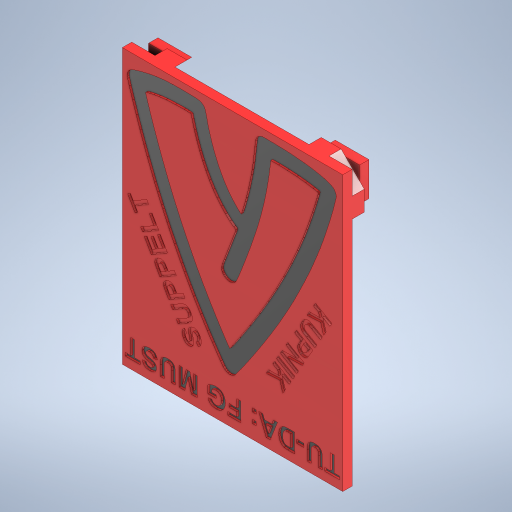
# Autodesk Inventor part: Battery_Cover
Saved by Autodesk Inventor 2023.3 (Build 273359000, 359)
## iProperties
Created: 2024-05-31
Part Number: Battery_Cover
Material: Generic
Document SubType Name: Modeling
Designer: Sven
Density: 1 g/cm^3
Appearance: Light Red
Author: Sven
Autodesk Inventor part; units mm, degrees
ref_plane "YZ Plane" through (0, 0, 0) normal (1, 0, 0) x (0, 1, 0)
ref_plane "XZ Plane" through (0, 0, 0) normal (0, 1, 0) x (-1, 0, 0)
ref_plane "XY Plane" through (0, 0, 0) normal (0, 0, 1) x (1, 0, 0)
sketch "Sketch1" plane through (0, 0, 0) normal (0, 0, 1) x (1, 0, 0)
  line L0 (1.45, 1.25) -> (1.45, -57.25) projected
  arc A0 (1.25, -57.45) -> (1.45, -57.25) centre (1.25, -57.25) ccw projected
  line L1 (1.25, -57.45) -> (-45.75, -57.45) projected
  arc A1 (-45.95, -57.25) -> (-45.75, -57.45) centre (-45.75, -57.25) ccw projected
  line L2 (-45.95, -57.25) -> (-45.95, 1.25) projected
  arc A2 (-45.75, 1.45) -> (-45.95, 1.25) centre (-45.75, 1.25) ccw projected
  line L3 (-45.75, 1.45) -> (1.25, 1.45) projected
  arc A3 (1.45, 1.25) -> (1.25, 1.45) centre (1.25, 1.25) ccw projected
  arc A4 (-45.75, 3.25) -> (-47.75, 1.25) centre (-45.75, 1.25) ccw projected
  line L4 (-47.75, -57.25) -> (-47.75, 1.25) projected
  arc A5 (-47.75, -57.25) -> (-45.75, -59.25) centre (-45.75, -57.25) ccw projected
  line L5 (1.25, -59.25) -> (-45.75, -59.25) projected
  arc A6 (1.25, -59.25) -> (3.25, -57.25) centre (1.25, -57.25) ccw projected
  line L6 (3.25, 1.25) -> (3.25, -57.25) projected
  arc A7 (3.25, 1.25) -> (1.25, 3.25) centre (1.25, 1.25) ccw projected
  line L7 (-45.75, 3.25) -> (1.25, 3.25) projected
  line L8 (1.25, 1.25) -> (-45.75, 1.25)
  line L9 (-45.75, 1.25) -> (-45.75, -57.25)
  line L10 (-45.75, -57.25) -> (1.25, -57.25)
  line L11 (1.25, -57.25) -> (1.25, 1.25)
  point P0 (0, 0)
  dimension "d0" = 0.2
  constraints: 8 end point, 23 other
  measures "d0" radius of A3
extrude "Extrusion1" add sketch "Sketch1" along normal blind 2 contours L11 L10 L9 L8
sketch "Sketch2" plane through (0, 0, 0) normal (0, 0, -1) x (-1, 0, 0)
  line L0 (-1.45, -3.05) -> (3.05, 1.45) projected
  line L1 (41.45, 1.45) -> (45.95, -3.05) projected
  line L2 (-1.45, 1.25) -> (-1.45, -57.25) projected
  arc A0 (-1.45, -57.25) -> (-1.25, -57.45) centre (-1.25, -57.25) ccw projected
  line L3 (-1.25, -57.45) -> (45.75, -57.45) projected
  arc A1 (45.75, -57.45) -> (45.95, -57.25) centre (45.75, -57.25) ccw projected
  line L4 (45.95, -57.25) -> (45.95, 1.25) projected
  arc A2 (45.95, 1.25) -> (45.75, 1.45) centre (45.75, 1.25) ccw projected
  line L5 (45.75, 1.45) -> (-1.25, 1.45) projected
  arc A3 (-1.25, 1.45) -> (-1.45, 1.25) centre (-1.25, 1.25) ccw projected
  arc A4 (47.75, 1.25) -> (45.75, 3.25) centre (45.75, 1.25) ccw projected
  line L6 (47.75, -57.25) -> (47.75, 1.25) projected
  arc A5 (45.75, -59.25) -> (47.75, -57.25) centre (45.75, -57.25) ccw projected
  line L7 (-1.25, -59.25) -> (45.75, -59.25) projected
  arc A6 (-3.25, -57.25) -> (-1.25, -59.25) centre (-1.25, -57.25) ccw projected
  line L8 (-3.25, 1.25) -> (-3.25, -57.25) projected
  arc A7 (-1.25, 3.25) -> (-3.25, 1.25) centre (-1.25, 1.25) ccw projected
  line L9 (45.75, 3.25) -> (-1.25, 3.25) projected
  line L10 (40.6015, 1.45) -> (45.95, -3.8985)
  line L11 (45.95, -8.1412) -> (36.3588, 1.45)
  line L12 (3.8985, 1.45) -> (-1.45, -3.8985)
  line L13 (-1.45, -8.1412) -> (8.1412, 1.45)
  line L14 (45.75, 1.25) -> (45.75, -57.25) projected
  line L15 (45.75, -57.25) -> (-1.25, -57.25) projected
  line L16 (-1.25, -57.25) -> (-1.25, 1.25) projected
  line L17 (-1.25, 1.25) -> (45.75, 1.25) projected
  point P0 (0, 0)
  point P1 (3.05, 1.45)
  point P2 (7.9412, 1.25)
  point P3 (3.6985, 1.25)
  point P4 (-1.25, -3.6985)
  point P5 (-1.25, -7.9412)
  point P6 (40.8015, 1.25)
  point P7 (36.5588, 1.25)
  point P8 (45.75, -7.9412)
  point P9 (45.75, -3.6985)
  dimension "d3" = 0.6
  dimension "d4" = 0.6
  dimension "d5" = 3
  dimension "d6" = 3
  constraints: 8 end point, 8 point on line, 3 parallel, 2 other
  measures "d4" distance between parallel lines of L10 L1
  measures "d5" distance between parallel lines of L11 L10
  measures "d6" distance between parallel lines of L13 L12
extrude "Extrusion2" add sketch "Sketch2" along normal blind 2.6 contours L12 L17 L13 L16 | L17 L10 L14 L11
sketch "Sketch3" plane through (0, 0, -2.6) normal (0, 0, -1) x (-1, 0, 0)
  line L0 (45.75, 1.25) -> (45.75, -57.25) projected
  line L1 (45.75, -57.25) -> (-1.25, -57.25) projected
  line L2 (-1.25, -57.25) -> (-1.25, 1.25) projected
  line L3 (-1.25, 1.25) -> (45.75, 1.25) projected
  line L4 (7.9412, 1.25) -> (-1.25, -7.9412) projected
  line L5 (36.5588, 1.25) -> (45.75, -7.9412) projected
  line L6 (44.75, 0.25) -> (44.75, -56.25)
  line L7 (44.75, -56.25) -> (-0.25, -56.25)
  line L8 (-0.25, -56.25) -> (-0.25, 0.25)
  line L9 (-0.25, 0.25) -> (44.75, 0.25)
  point P0 (0, 0)
  point P1 (37.5588, 0.25)
  point P2 (44.75, -6.9412)
  point P3 (6.9412, 0.25)
  point P4 (-0.25, -6.9412)
  dimension "d11" = 1
  constraints: 8 end point, 3 other
  measures "d11" distance between parallel lines of L3 L9
extrude "Extrusion3" add sketch "Sketch3" along normal blind 2 contours L5 L9 L6 | L4 L8 L9
sketch "Sketch6" plane through (-45.75, -57.25, 0) normal (0, -1, 0) x (1, 0, 0)
  circle A0 centre (23.5, -4) radius 2
  circle A1 centre (23.5, -4) radius 4
  line L0 (37.8088, 0) -> (9.1912, 0) projected
  line L1 (19.5, 0) -> (19.5, -4)
  line L2 (0, 0) -> (47, 0) projected
  line L3 (47, 0) -> (47, 2) projected
  line L4 (0, 2) -> (47, 2) projected
  line L5 (0, 0) -> (0, 2) projected
  line L6 (27.5, -4) -> (27.5, 0)
  point P0 (45.75, 0)
  point P1 (23.5, 0)
  point P2 (23.5, 0)
  dimension "d12" = 4
  dimension "d13" = 8
  dimension "d14" = 4
  constraints: 4 end point, 3 point on line, 2 centre point, 2 perpendicular, 2 point on circle, 1 coincident, 1 horizontal alignment, 1 midpoint, 1 tangent, 1 vertical alignment
  measures "d12" diameter of A0
  measures "d13" diameter of A1
  measures "d14" distance from line of A0.centre L1
extrude "Extrusion4" add sketch "Sketch6" against normal blind 4 contours A1 | L1 L0 A1 | A1 L0 L6
sketch "Sketch7" plane through (0, 0, 2) normal (0, 0, 1) x (1, 0, 0)
  line L0 (-22.4218, -47.5937) -> (-22.1301, -47.4796)
  line L1 (-22.1301, -47.4796) -> (-21.877, -47.3459)
  line L2 (-21.877, -47.3459) -> (-21.7005, -47.1679)
  line L3 (-21.7005, -47.1679) -> (-21.3935, -46.7869)
  line L4 (-21.3935, -46.7869) -> (-20.4434, -45.4927)
  line L5 (-20.4434, -45.4927) -> (-19.1363, -43.6172)
  line L6 (-19.1363, -43.6172) -> (-17.582, -41.3146)
  line L7 (-17.582, -41.3146) -> (-15.6954, -38.4287)
  line L8 (-15.6954, -38.4287) -> (-13.9508, -35.6534)
  line L9 (-13.9508, -35.6534) -> (-12.3797, -33.0397)
  line L10 (-12.3797, -33.0397) -> (-11.0135, -30.6387)
  line L11 (-11.0135, -30.6387) -> (-10.5549, -29.8053)
  line L12 (-10.5549, -29.8053) -> (-10.1581, -29.0883)
  line L13 (-10.1581, -29.0883) -> (-9.2164, -27.3215)
  line L14 (-9.2164, -27.3215) -> (-8.0832, -25.0645)
  line L15 (-8.0832, -25.0645) -> (-6.8816, -22.5677)
  line L16 (-6.8816, -22.5677) -> (-5.7346, -20.0818)
  line L17 (-5.7346, -20.0818) -> (-5.0005, -18.3637)
  line L18 (-5.0005, -18.3637) -> (-4.1712, -16.3115)
  line L19 (-4.1712, -16.3115) -> (-3.5332, -14.6843)
  line L20 (-3.5332, -14.6843) -> (-2.8607, -12.8431)
  line L21 (-2.8607, -12.8431) -> (-2.0725, -10.4909)
  line L22 (-2.0725, -10.4909) -> (-1.3096, -8.0625)
  line L23 (-1.3096, -8.0625) -> (-0.7131, -5.9927)
  line L24 (-0.7131, -5.9927) -> (-0.178, -3.8718)
  line L25 (-0.178, -3.8718) -> (-0.1259, -3.4434)
  line L26 (-0.1259, -3.4434) -> (-0.1633, -3.1565)
  line L27 (-0.1633, -3.1565) -> (-0.307, -2.75)
  line L28 (-0.307, -2.75) -> (-0.5289, -2.4081)
  line L29 (-0.5289, -2.4081) -> (-0.8313, -2.1281)
  line L30 (-0.8313, -2.1281) -> (-1.2166, -1.9072)
  line L31 (-1.2166, -1.9072) -> (-1.8713, -1.6499)
  line L32 (-1.8713, -1.6499) -> (-2.6489, -1.4111)
  line L33 (-2.6489, -1.4111) -> (-3.5464, -1.1913)
  line L34 (-3.5464, -1.1913) -> (-4.5606, -0.991)
  line L35 (-4.5606, -0.991) -> (-5.6885, -0.8107)
  line L36 (-5.6885, -0.8107) -> (-6.927, -0.6511)
  line L37 (-6.927, -0.6511) -> (-9.7234, -0.396)
  line L38 (-9.7234, -0.396) -> (-11.2918, -0.3192)
  line L39 (-11.2918, -0.3192) -> (-13.2274, -0.2646)
  line L40 (-13.2274, -0.2646) -> (-14.9519, -0.244)
  line L41 (-14.9519, -0.244) -> (-15.8868, -0.2692)
  line L42 (-15.8868, -0.2692) -> (-16.2879, -0.3827)
  line L43 (-16.2879, -0.3827) -> (-16.6498, -0.5883)
  line L44 (-16.6498, -0.5883) -> (-16.9519, -0.8711)
  line L45 (-16.9519, -0.8711) -> (-17.1736, -1.2157)
  line L46 (-17.1736, -1.2157) -> (-17.2762, -1.4809)
  line L47 (-17.2762, -1.4809) -> (-17.3555, -1.8239)
  line L48 (-17.3555, -1.8239) -> (-17.5001, -3.0559)
  line L49 (-17.5001, -3.0559) -> (-17.8576, -6.0814)
  line L50 (-17.8576, -6.0814) -> (-18.0686, -7.5036)
  line L51 (-18.0686, -7.5036) -> (-18.2552, -8.5327)
  line L52 (-18.2552, -8.5327) -> (-18.4522, -9.5249)
  line L53 (-18.4522, -9.5249) -> (-18.8507, -11.3902)
  line L54 (-18.8507, -11.3902) -> (-19.3272, -13.3349)
  line L55 (-19.3272, -13.3349) -> (-19.5659, -14.2081)
  line L56 (-19.5659, -14.2081) -> (-20.1091, -16.0832)
  line L57 (-20.1091, -16.0832) -> (-20.3018, -16.6302)
  line L58 (-20.3018, -16.6302) -> (-20.413, -16.8274)
  line L59 (-20.413, -16.8274) -> (-20.5442, -16.7465)
  line L60 (-20.5442, -16.7465) -> (-20.7913, -16.5264)
  line L61 (-20.7913, -16.5264) -> (-21.5056, -15.8033)
  line L62 (-21.5056, -15.8033) -> (-22.3007, -14.9285)
  line L63 (-22.3007, -14.9285) -> (-22.9214, -14.1719)
  line L64 (-22.9214, -14.1719) -> (-23.5334, -13.2933)
  line L65 (-23.5334, -13.2933) -> (-24.1204, -12.3504)
  line L66 (-24.1204, -12.3504) -> (-24.6801, -11.3485)
  line L67 (-24.6801, -11.3485) -> (-25.2099, -10.2927)
  line L68 (-25.2099, -10.2927) -> (-25.7073, -9.1882)
  line L69 (-25.7073, -9.1882) -> (-26.1699, -8.0404)
  line L70 (-26.1699, -8.0404) -> (-26.595, -6.8544)
  line L71 (-26.595, -6.8544) -> (-26.9804, -5.6355)
  line L72 (-26.9804, -5.6355) -> (-27.3013, -4.564)
  line L73 (-27.3013, -4.564) -> (-27.4992, -3.787)
  line L74 (-27.4992, -3.787) -> (-27.8233, -2.3169)
  line L75 (-27.8233, -2.3169) -> (-28.0099, -1.5913)
  line L76 (-28.0099, -1.5913) -> (-28.1897, -1.1074)
  line L77 (-28.1897, -1.1074) -> (-28.3778, -0.8494)
  line L78 (-28.3778, -0.8494) -> (-28.627, -0.6256)
  line L79 (-28.627, -0.6256) -> (-28.9225, -0.447)
  line L80 (-28.9225, -0.447) -> (-29.2497, -0.3244)
  line L81 (-29.2497, -0.3244) -> (-29.7226, -0.2539)
  line L82 (-29.7226, -0.2539) -> (-30.4996, -0.2007)
  line L83 (-30.4996, -0.2007) -> (-32.6371, -0.1486)
  line L84 (-32.6371, -0.1486) -> (-35.0058, -0.1721)
  line L85 (-35.0058, -0.1721) -> (-36.9491, -0.2755)
  line L86 (-36.9491, -0.2755) -> (-38.4208, -0.4624)
  line L87 (-38.4208, -0.4624) -> (-39.9715, -0.7419)
  line L88 (-39.9715, -0.7419) -> (-41.5045, -1.0942)
  line L89 (-41.5045, -1.0942) -> (-42.9231, -1.4994)
  line L90 (-42.9231, -1.4994) -> (-43.6496, -1.7694)
  line L91 (-43.6496, -1.7694) -> (-43.9195, -1.9088)
  line L92 (-43.9195, -1.9088) -> (-44.1379, -2.0598)
  line L93 (-44.1379, -2.0598) -> (-44.3128, -2.229)
  line L94 (-44.3128, -2.229) -> (-44.4522, -2.4229)
  line L95 (-44.4522, -2.4229) -> (-44.5641, -2.6479)
  line L96 (-44.5641, -2.6479) -> (-44.6566, -2.9108)
  line L97 (-44.6566, -2.9108) -> (-44.7035, -3.0894)
  line L98 (-44.7035, -3.0894) -> (-44.7221, -3.2777)
  line L99 (-44.7221, -3.2777) -> (-44.7002, -3.5245)
  line L100 (-44.7002, -3.5245) -> (-44.6258, -3.8785)
  line L101 (-44.6258, -3.8785) -> (-44.2713, -5.1033)
  line L102 (-44.2713, -5.1033) -> (-43.5625, -7.3421)
  line L103 (-43.5625, -7.3421) -> (-42.7838, -9.7208)
  line L104 (-42.7838, -9.7208) -> (-41.9684, -12.1044)
  line L105 (-41.9684, -12.1044) -> (-41.1688, -14.3422)
  line L106 (-41.1688, -14.3422) -> (-40.4377, -16.2837)
  line L107 (-40.4377, -16.2837) -> (-38.8935, -20.2009)
  line L108 (-38.8935, -20.2009) -> (-38.2563, -21.709)
  line L109 (-38.2563, -21.709) -> (-37.4187, -23.6409)
  line L110 (-37.4187, -23.6409) -> (-37.1475, -24.2505)
  line L111 (-37.1475, -24.2505) -> (-36.226, -26.2613)
  line L112 (-36.226, -26.2613) -> (-35.7981, -27.1981)
  line L113 (-35.7981, -27.1981) -> (-34.6606, -29.5092)
  line L114 (-34.6606, -29.5092) -> (-33.2215, -32.3453)
  line L115 (-33.2215, -32.3453) -> (-32.5435, -33.6153)
  line L116 (-32.5435, -33.6153) -> (-31.4901, -35.5203)
  line L117 (-31.4901, -35.5203) -> (-30.5845, -37.1291)
  line L118 (-30.5845, -37.1291) -> (-29.0661, -39.6601)
  line L119 (-29.0661, -39.6601) -> (-27.6238, -41.9849)
  line L120 (-27.6238, -41.9849) -> (-26.5469, -43.6165)
  line L121 (-26.5469, -43.6165) -> (-24.8199, -46.165)
  line L122 (-24.8199, -46.165) -> (-24.2589, -46.9183)
  line L123 (-24.2589, -46.9183) -> (-23.9183, -47.2977)
  line L124 (-23.9183, -47.2977) -> (-23.6107, -47.4814)
  line L125 (-23.6107, -47.4814) -> (-23.2487, -47.6118)
  line L126 (-23.2487, -47.6118) -> (-22.8119, -47.6911)
  line L127 (-22.8119, -47.6911) -> (-22.4218, -47.5937)
  line L128 (-23.6277, -41.771) -> (-25.2618, -39.2361)
  line L129 (-25.2618, -39.2361) -> (-26.8845, -36.5814)
  line L130 (-26.8845, -36.5814) -> (-28.4419, -33.8972)
  line L131 (-28.4419, -33.8972) -> (-29.8805, -31.2737)
  line L132 (-29.8805, -31.2737) -> (-31.4525, -28.1832)
  line L133 (-31.4525, -28.1832) -> (-32.9151, -25.2015)
  line L134 (-32.9151, -25.2015) -> (-34.7034, -21.239)
  line L135 (-34.7034, -21.239) -> (-36.0125, -18.0974)
  line L136 (-36.0125, -18.0974) -> (-36.9476, -15.7162)
  line L137 (-36.9476, -15.7162) -> (-37.9077, -13.1798)
  line L138 (-37.9077, -13.1798) -> (-38.9612, -10.2393)
  line L139 (-38.9612, -10.2393) -> (-40.1298, -6.7391)
  line L140 (-40.1298, -6.7391) -> (-40.7988, -4.5596)
  line L141 (-40.7988, -4.5596) -> (-40.7415, -4.5066)
  line L142 (-40.7415, -4.5066) -> (-40.5772, -4.4392)
  line L143 (-40.5772, -4.4392) -> (-39.9732, -4.2725)
  line L144 (-39.9732, -4.2725) -> (-39.0775, -4.081)
  line L145 (-39.0775, -4.081) -> (-37.981, -3.8866)
  line L146 (-37.981, -3.8866) -> (-36.4336, -3.7221)
  line L147 (-36.4336, -3.7221) -> (-34.4459, -3.6115)
  line L148 (-34.4459, -3.6115) -> (-32.5787, -3.5761)
  line L149 (-32.5787, -3.5761) -> (-31.8655, -3.5932)
  line L150 (-31.8655, -3.5932) -> (-31.3928, -3.637)
  line L151 (-31.3928, -3.637) -> (-31.0753, -3.6932)
  line L152 (-31.0753, -3.6932) -> (-30.8594, -4.5651)
  line L153 (-30.8594, -4.5651) -> (-30.3916, -6.297)
  line L154 (-30.3916, -6.297) -> (-29.8599, -7.976)
  line L155 (-29.8599, -7.976) -> (-29.2685, -9.5929)
  line L156 (-29.2685, -9.5929) -> (-28.6213, -11.1387)
  line L157 (-28.6213, -11.1387) -> (-27.9225, -12.6044)
  line L158 (-27.9225, -12.6044) -> (-27.176, -13.981)
  line L159 (-27.176, -13.981) -> (-26.386, -15.2594)
  line L160 (-26.386, -15.2594) -> (-25.5564, -16.4306)
  line L161 (-25.5564, -16.4306) -> (-24.6896, -17.4843)
  line L162 (-24.6896, -17.4843) -> (-23.7502, -18.4804)
  line L163 (-23.7502, -18.4804) -> (-22.8212, -19.3365)
  line L164 (-22.8212, -19.3365) -> (-21.9856, -19.9704)
  line L165 (-21.9856, -19.9704) -> (-21.5608, -20.2516)
  line L166 (-21.5608, -20.2516) -> (-21.57, -20.4474)
  line L167 (-21.57, -20.4474) -> (-21.6915, -20.8469)
  line L168 (-21.6915, -20.8469) -> (-24.085, -27.1739)
  line L169 (-24.085, -27.1739) -> (-24.4169, -28.0733)
  line L170 (-24.4169, -28.0733) -> (-24.5759, -28.6748)
  line L171 (-24.5759, -28.6748) -> (-24.5969, -28.9035)
  line L172 (-24.5969, -28.9035) -> (-24.5823, -29.1053)
  line L173 (-24.5823, -29.1053) -> (-24.4566, -29.4922)
  line L174 (-24.4566, -29.4922) -> (-24.317, -29.7331)
  line L175 (-24.317, -29.7331) -> (-24.1315, -29.9526)
  line L176 (-24.1315, -29.9526) -> (-23.91, -30.1455)
  line L177 (-23.91, -30.1455) -> (-23.6623, -30.3063)
  line L178 (-23.6623, -30.3063) -> (-23.3982, -30.4294)
  line L179 (-23.3982, -30.4294) -> (-23.1275, -30.5095)
  line L180 (-23.1275, -30.5095) -> (-22.86, -30.5412)
  line L181 (-22.86, -30.5412) -> (-22.6055, -30.5189)
  line L182 (-22.6055, -30.5189) -> (-22.2834, -30.412)
  line L183 (-22.2834, -30.412) -> (-21.9629, -30.2372)
  line L184 (-21.9629, -30.2372) -> (-21.6814, -30.0188)
  line L185 (-21.6814, -30.0188) -> (-21.476, -29.781)
  line L186 (-21.476, -29.781) -> (-21.049, -28.8468)
  line L187 (-21.049, -28.8468) -> (-20.2895, -26.9559)
  line L188 (-20.2895, -26.9559) -> (-19.3541, -24.5092)
  line L189 (-19.3541, -24.5092) -> (-18.3995, -21.9074)
  line L190 (-18.3995, -21.9074) -> (-17.1916, -18.3544)
  line L191 (-17.1916, -18.3544) -> (-16.6761, -16.6836)
  line L192 (-16.6761, -16.6836) -> (-16.2062, -15.0415)
  line L193 (-16.2062, -15.0415) -> (-15.536, -12.4011)
  line L194 (-15.536, -12.4011) -> (-14.9703, -9.7343)
  line L195 (-14.9703, -9.7343) -> (-14.5074, -7.0322)
  line L196 (-14.5074, -7.0322) -> (-14.1457, -4.2862)
  line L197 (-14.1457, -4.2862) -> (-14.0877, -3.7702)
  line L198 (-14.0877, -3.7702) -> (-12.4612, -3.7776)
  line L199 (-12.4612, -3.7776) -> (-10.5503, -3.8309)
  line L200 (-10.5503, -3.8309) -> (-8.5668, -3.9644)
  line L201 (-8.5668, -3.9644) -> (-6.6852, -4.1631)
  line L202 (-6.6852, -4.1631) -> (-5.08, -4.412)
  line L203 (-5.08, -4.412) -> (-4.187, -4.5813)
  line L204 (-4.187, -4.5813) -> (-4.0474, -4.631)
  line L205 (-4.0474, -4.631) -> (-3.9799, -4.7265)
  line L206 (-3.9799, -4.7265) -> (-3.9797, -4.886)
  line L207 (-3.9797, -4.886) -> (-4.0421, -5.1276)
  line L208 (-4.0421, -5.1276) -> (-4.2861, -5.953)
  line L209 (-4.2861, -5.953) -> (-4.5191, -6.7468)
  line L210 (-4.5191, -6.7468) -> (-4.7106, -7.3818)
  line L211 (-4.7106, -7.3818) -> (-5.2254, -9.0203)
  line L212 (-5.2254, -9.0203) -> (-5.8807, -10.9641)
  line L213 (-5.8807, -10.9641) -> (-6.5795, -12.9326)
  line L214 (-6.5795, -12.9326) -> (-7.2246, -14.6453)
  line L215 (-7.2246, -14.6453) -> (-8.4936, -17.7356)
  line L216 (-8.4936, -17.7356) -> (-9.8713, -20.8205)
  line L217 (-9.8713, -20.8205) -> (-11.364, -23.9116)
  line L218 (-11.364, -23.9116) -> (-12.9781, -27.0209)
  line L219 (-12.9781, -27.0209) -> (-14.7199, -30.1599)
  line L220 (-14.7199, -30.1599) -> (-16.5956, -33.3405)
  line L221 (-16.5956, -33.3405) -> (-18.6116, -36.5743)
  line L222 (-18.6116, -36.5743) -> (-20.7741, -39.8732)
  line L223 (-20.7741, -39.8732) -> (-22.3894, -42.2553)
  line L224 (-22.3894, -42.2553) -> (-22.7302, -42.7247)
  line L225 (-22.7302, -42.7247) -> (-22.862, -42.8594)
  line L226 (-22.862, -42.8594) -> (-23.6277, -41.771)
  line L227 (-21.3916, -15.9146) -> (-21.8281, -15.4781)
  line L228 (-21.8281, -15.4781) -> (-21.3916, -15.9146)
  line L229 (-21.3916, -15.9146) -> (-20.955, -16.3512)
  line L230 (-20.955, -16.3512) -> (-21.3916, -15.9146)
  point P0 (0, 0)
  constraints: 462 end point
extrude "Extrusion5" cut sketch "Sketch7" against normal blind 0.4
sketch "Sketch8" plane through (0, 0, 2) normal (0, 0, 1) x (1, 0, 0)
  line L0 (1.7615, -55.4851) -> (-46.3064, -55.4851) construction
  line L1 (-46.3064, -55.4851) -> (-46.3064, -49.2125) construction
  line L2 (-46.3064, -49.2125) -> (1.7615, -49.2125) construction
  line L3 (1.7615, -49.2125) -> (1.7615, -55.4851) construction
  line L4 (-0.6078, -51.418) -> (-0.6078, -54.7412)
  line L5 (-0.6078, -54.7412) -> (0.5782, -54.7412)
  line L6 (0.5782, -54.7412) -> (0.5782, -55.418)
  line L7 (0.5782, -55.418) -> (-2.5987, -55.418)
  line L8 (-2.5987, -55.418) -> (-2.5987, -54.7412)
  line L9 (-2.5987, -54.7412) -> (-1.4157, -54.7412)
  line L10 (-1.4157, -54.7412) -> (-1.4157, -51.418)
  line L11 (-1.4157, -51.418) -> (-0.6078, -51.418)
  line L12 (-3.117, -55.418) -> (-3.9249, -55.418)
  line L13 (-3.9249, -55.418) -> (-3.9249, -53.2503)
  spline S0 degree 2 poles (-3.9249, -53.2503) (-3.9249, -52.7351) (-3.9554, -52.5826) knots 0 0 0 1 1 1
  spline S1 degree 2 poles (-3.9554, -52.5826) (-4.0072, -52.3387) (-4.3975, -52.04) (-4.7359, -52.04) knots 0 0 0 1 2 2 2
  spline S2 degree 2 poles (-4.7359, -52.04) (-5.0773, -52.04) (-5.4279, -52.3204) (-5.4981, -52.729) (-5.4981, -53.2046) knots 0 0 0 1 2 3 3 3
  line L14 (-5.4981, -53.2046) -> (-5.4981, -55.418)
  line L15 (-5.4981, -55.418) -> (-6.306, -55.418)
  line L16 (-6.306, -55.418) -> (-6.306, -53.3174)
  spline S3 degree 2 poles (-6.306, -53.3174) (-6.306, -52.5979) (-6.1749, -52.0034) (-5.8243, -51.5948) (-5.2328, -51.3509) (-4.7603, -51.3509) knots 0 0 0 1 2 3 4 4 4
  spline S4 degree 2 poles (-4.7603, -51.3509) (-4.1871, -51.3509) (-3.5956, -51.6162) (-3.2511, -52.0369) (-3.1962, -52.2717) knots 0 0 0 1 2 3 3 3
  spline S5 degree 2 poles (-3.1962, -52.2717) (-3.117, -52.6131) (-3.117, -53.2839) knots 0 0 0 1 1 1
  line L17 (-3.117, -53.2839) -> (-3.117, -55.418)
  line L18 (-7.0651, -52.4851) -> (-7.0651, -53.2534)
  line L19 (-7.0651, -53.2534) -> (-8.5712, -53.2534)
  line L20 (-8.5712, -53.2534) -> (-8.5712, -52.4851)
  line L21 (-8.5712, -52.4851) -> (-7.0651, -52.4851)
  line L22 (-9.0133, -55.418) -> (-10.492, -55.418)
  spline S6 degree 2 poles (-10.492, -55.418) (-10.992, -55.418) (-11.2542, -55.3418) knots 0 0 0 1 1 1
  spline S7 degree 2 poles (-11.2542, -55.3418) (-11.6048, -55.2381) (-12.1078, -54.7076) (-12.37, -53.9424) (-12.37, -53.3784) knots 0 0 0 1 2 3 3 3
  spline S8 degree 2 poles (-12.37, -53.3784) (-12.37, -52.8845) (-12.2481, -52.5278) knots 0 0 0 1 1 1
  spline S9 degree 2 poles (-12.2481, -52.5278) (-12.0956, -52.0918) (-11.8182, -51.8204) knots 0 0 0 1 1 1
  spline S10 degree 2 poles (-11.8182, -51.8204) (-11.6078, -51.6162) (-11.2511, -51.5034) knots 0 0 0 1 1 1
  spline S11 degree 2 poles (-11.2511, -51.5034) (-10.9828, -51.418) (-10.5346, -51.418) knots 0 0 0 1 1 1
  line L23 (-10.5346, -51.418) -> (-9.0133, -51.418)
  line L24 (-9.0133, -51.418) -> (-9.0133, -55.418)
  line L25 (-9.8212, -54.7412) -> (-9.8212, -52.0948)
  line L26 (-9.8212, -52.0948) -> (-10.4249, -52.0948)
  spline S12 degree 2 poles (-10.4249, -52.0948) (-10.7664, -52.0948) (-10.9157, -52.1345) knots 0 0 0 1 1 1
  spline S13 degree 2 poles (-10.9157, -52.1345) (-11.1139, -52.1832) (-11.3731, -52.415) (-11.5377, -52.9546) (-11.5377, -53.418) knots 0 0 0 1 2 3 3 3
  spline S14 degree 2 poles (-11.5377, -53.418) (-11.5377, -53.8814) (-11.3731, -54.3753) (-11.0773, -54.6528) (-10.8517, -54.7015) knots 0 0 0 1 2 3 3 3
  spline S15 degree 2 poles (-10.8517, -54.7015) (-10.681, -54.7412) (-10.184, -54.7412) knots 0 0 0 1 1 1
  line L27 (-10.184, -54.7412) -> (-9.8212, -54.7412)
  line L28 (-16.6596, -51.418) -> (-15.7816, -51.418)
  line L29 (-15.7816, -51.418) -> (-15.434, -52.3265)
  line L30 (-15.434, -52.3265) -> (-13.8365, -52.3265)
  line L31 (-13.8365, -52.3265) -> (-13.5042, -51.418)
  line L32 (-13.5042, -51.418) -> (-12.6475, -51.418)
  line L33 (-12.6475, -51.418) -> (-14.2023, -55.418)
  line L34 (-14.2023, -55.418) -> (-15.0621, -55.418)
  line L35 (-15.0621, -55.418) -> (-16.6596, -51.418)
  line L36 (-15.1749, -53.0034) -> (-14.6231, -54.4851)
  line L37 (-14.6231, -54.4851) -> (-14.0804, -53.0034)
  line L38 (-14.0804, -53.0034) -> (-15.1749, -53.0034)
  line L39 (-17.2298, -51.418) -> (-17.2298, -52.1863)
  line L40 (-17.2298, -52.1863) -> (-17.9981, -52.1863)
  line L41 (-17.9981, -52.1863) -> (-17.9981, -51.418)
  line L42 (-17.9981, -51.418) -> (-17.2298, -51.418)
  line L43 (-17.2298, -53.5491) -> (-17.2298, -54.3174)
  line L44 (-17.2298, -54.3174) -> (-17.9981, -54.3174)
  line L45 (-17.9981, -54.3174) -> (-17.9981, -53.5491)
  line L46 (-17.9981, -53.5491) -> (-17.2298, -53.5491)
  line L47 (-20.5042, -51.418) -> (-20.5042, -55.418)
  line L48 (-20.5042, -55.418) -> (-23.2511, -55.418)
  line L49 (-23.2511, -55.418) -> (-23.2511, -54.7412)
  line L50 (-23.2511, -54.7412) -> (-21.3121, -54.7412)
  line L51 (-21.3121, -54.7412) -> (-21.3121, -53.796)
  line L52 (-21.3121, -53.796) -> (-22.9859, -53.796)
  line L53 (-22.9859, -53.796) -> (-22.9859, -53.1192)
  line L54 (-22.9859, -53.1192) -> (-21.3121, -53.1192)
  line L55 (-21.3121, -53.1192) -> (-21.3121, -51.418)
  line L56 (-21.3121, -51.418) -> (-20.5042, -51.418)
  line L57 (-25.7785, -52.8845) -> (-25.7785, -53.5613)
  line L58 (-25.7785, -53.5613) -> (-27.5194, -53.5613)
  line L59 (-27.5194, -53.5613) -> (-27.5194, -51.9698)
  spline S16 degree 2 poles (-27.5194, -51.9698) (-27.2664, -51.7229) (-26.3029, -51.3509) (-25.809, -51.3509) knots 0 0 0 1 2 2 2
  spline S17 degree 2 poles (-25.809, -51.3509) (-25.181, -51.3509) (-24.2481, -51.8784) (-23.7785, -52.857) (-23.7785, -53.4302) knots 0 0 0 1 2 3 3 3
  spline S18 degree 2 poles (-23.7785, -53.4302) (-23.7785, -54.0552) (-24.3029, -55.0278) (-24.806, -55.2869) knots 0 0 0 1 2 2 2
  spline S19 degree 2 poles (-24.806, -55.2869) (-25.1932, -55.4851) (-25.7664, -55.4851) knots 0 0 0 1 1 1
  spline S20 degree 2 poles (-25.7664, -55.4851) (-26.5103, -55.4851) (-27.3487, -54.8601) (-27.4676, -54.3082) knots 0 0 0 1 2 2 2
  line L60 (-27.4676, -54.3082) -> (-26.6657, -54.1589)
  spline S21 degree 2 poles (-26.6657, -54.1589) (-26.5804, -54.4546) (-26.1139, -54.796) (-25.7664, -54.796) knots 0 0 0 1 2 2 2
  spline S22 degree 2 poles (-25.7664, -54.796) (-25.2359, -54.796) (-24.6109, -54.1253) (-24.6109, -53.4637) knots 0 0 0 1 2 2 2
  spline S23 degree 2 poles (-24.6109, -53.4637) (-24.6109, -52.7534) (-25.245, -52.04) (-25.7572, -52.04) knots 0 0 0 1 2 2 2
  spline S24 degree 2 poles (-25.7572, -52.04) (-26.0103, -52.04) (-26.5194, -52.2381) (-26.7023, -52.3784) knots 0 0 0 1 2 2 2
  line L61 (-26.7023, -52.3784) -> (-26.7023, -52.8845)
  line L62 (-26.7023, -52.8845) -> (-25.7785, -52.8845)
  line L63 (-29.809, -51.418) -> (-29.809, -55.418)
  line L64 (-29.809, -55.418) -> (-31.0194, -55.418)
  line L65 (-31.0194, -55.418) -> (-31.742, -52.6893)
  line L66 (-31.742, -52.6893) -> (-32.4523, -55.418)
  line L67 (-32.4523, -55.418) -> (-33.6657, -55.418)
  line L68 (-33.6657, -55.418) -> (-33.6657, -51.418)
  line L69 (-33.6657, -51.418) -> (-32.9188, -51.418)
  line L70 (-32.9188, -51.418) -> (-32.9188, -54.5674)
  line L71 (-32.9188, -54.5674) -> (-32.1261, -51.418)
  line L72 (-32.1261, -51.418) -> (-31.3456, -51.418)
  line L73 (-31.3456, -51.418) -> (-30.559, -54.5674)
  line L74 (-30.559, -54.5674) -> (-30.556, -51.418)
  line L75 (-30.556, -51.418) -> (-29.809, -51.418)
  line L76 (-34.4676, -55.418) -> (-35.2755, -55.418)
  line L77 (-35.2755, -55.418) -> (-35.2755, -53.2503)
  spline S25 degree 2 poles (-35.2755, -53.2503) (-35.2755, -52.7351) (-35.306, -52.5826) knots 0 0 0 1 1 1
  spline S26 degree 2 poles (-35.306, -52.5826) (-35.3578, -52.3387) (-35.7481, -52.04) (-36.0865, -52.04) knots 0 0 0 1 2 2 2
  spline S27 degree 2 poles (-36.0865, -52.04) (-36.4279, -52.04) (-36.7786, -52.3204) (-36.8487, -52.729) (-36.8487, -53.2046) knots 0 0 0 1 2 3 3 3
  line L78 (-36.8487, -53.2046) -> (-36.8487, -55.418)
  line L79 (-36.8487, -55.418) -> (-37.6566, -55.418)
  line L80 (-37.6566, -55.418) -> (-37.6566, -53.3174)
  spline S28 degree 2 poles (-37.6566, -53.3174) (-37.6566, -52.5979) (-37.5255, -52.0034) (-37.1749, -51.5948) (-36.5834, -51.3509) (-36.1109, -51.3509) knots 0 0 0 1 2 3 4 4 4
  spline S29 degree 2 poles (-36.1109, -51.3509) (-35.5377, -51.3509) (-34.9462, -51.6162) (-34.6017, -52.0369) (-34.5468, -52.2717) knots 0 0 0 1 2 3 3 3
  spline S30 degree 2 poles (-34.5468, -52.2717) (-34.4676, -52.6131) (-34.4676, -53.2839) knots 0 0 0 1 1 1
  line L81 (-34.4676, -53.2839) -> (-34.4676, -55.418)
  line L82 (-38.3029, -52.7229) -> (-39.0895, -52.7991)
  spline S31 degree 2 poles (-39.0895, -52.7991) (-39.1596, -52.4028) (-39.5956, -52.0308) (-39.9615, -52.0308) knots 0 0 0 1 2 2 2
  spline S32 degree 2 poles (-39.9615, -52.0308) (-40.3517, -52.0308) (-40.7481, -52.3601) (-40.7481, -52.5826) knots 0 0 0 1 2 2 2
  spline S33 degree 2 poles (-40.7481, -52.5826) (-40.7481, -52.7259) (-40.5804, -52.9241) (-40.3731, -52.9973) knots 0 0 0 1 2 2 2
  spline S34 degree 2 poles (-40.3731, -52.9973) (-40.2328, -53.046) (-39.7267, -53.171) knots 0 0 0 1 1 1
  spline S35 degree 2 poles (-39.7267, -53.171) (-39.0773, -53.3326) (-38.8151, -53.5674) knots 0 0 0 1 1 1
  spline S36 degree 2 poles (-38.8151, -53.5674) (-38.4462, -53.8967) (-38.4462, -54.3692) knots 0 0 0 1 1 1
  spline S37 degree 2 poles (-38.4462, -54.3692) (-38.4462, -54.6771) (-38.7938, -55.2076) (-39.4462, -55.4851) (-39.9066, -55.4851) knots 0 0 0 1 2 3 3 3
  spline S38 degree 2 poles (-39.9066, -55.4851) (-40.6596, -55.4851) (-41.4218, -54.8265) (-41.4401, -54.2747) knots 0 0 0 1 2 2 2
  line L83 (-41.4401, -54.2747) -> (-40.6322, -54.2381)
  spline S39 degree 2 poles (-40.6322, -54.2381) (-40.5804, -54.546) (-40.2389, -54.8174) (-39.8975, -54.8174) knots 0 0 0 1 2 2 2
  spline S40 degree 2 poles (-39.8975, -54.8174) (-39.5438, -54.8174) (-39.3456, -54.6741) knots 0 0 0 1 1 1
  spline S41 degree 2 poles (-39.3456, -54.6741) (-39.2176, -54.5796) (-39.2176, -54.4241) knots 0 0 0 1 1 1
  spline S42 degree 2 poles (-39.2176, -54.4241) (-39.2176, -54.2839) (-39.3365, -54.1802) knots 0 0 0 1 1 1
  spline S43 degree 2 poles (-39.3365, -54.1802) (-39.492, -54.0521) (-40.6718, -53.7747) (-41.2359, -53.479) (-41.556, -52.9637) (-41.556, -52.5826) knots 0 0 0 1 2 3 4 4 4
  spline S44 degree 2 poles (-41.556, -52.5826) (-41.556, -52.2412) (-41.1749, -51.6406) (-40.4767, -51.3479) (-39.9554, -51.3479) knots 0 0 0 1 2 3 3 3
  spline S45 degree 2 poles (-39.9554, -51.3479) (-39.1962, -51.3479) (-38.3822, -52.0491) (-38.3029, -52.7229) knots 0 0 0 1 2 2 2
  line L84 (-43.1383, -51.418) -> (-43.1383, -54.7412)
  line L85 (-43.1383, -54.7412) -> (-41.9523, -54.7412)
  line L86 (-41.9523, -54.7412) -> (-41.9523, -55.418)
  line L87 (-41.9523, -55.418) -> (-45.1292, -55.418)
  line L88 (-45.1292, -55.418) -> (-45.1292, -54.7412)
  line L89 (-45.1292, -54.7412) -> (-43.9462, -54.7412)
  line L90 (-43.9462, -54.7412) -> (-43.9462, -51.418)
  line L91 (-43.9462, -51.418) -> (-43.1383, -51.418)
  point P0 (0, 0)
  constraints: 2 other
extrude "Extrusion6" cut sketch "Sketch8" against normal blind 0.4
sketch "Skizze9" plane through (0, 0, 2) normal (0, 0, 1) x (1, 0, 0)
  line L0 (-31.8282, -47.4448) -> (-44.7162, -25.1223) construction
  line L1 (-44.7162, -25.1223) -> (-41.194, -23.0887) construction
  line L2 (-41.194, -23.0887) -> (-28.306, -45.4113) construction
  line L3 (-28.306, -45.4113) -> (-31.8282, -47.4448) construction
  line L4 (0.2162, -25.1223) -> (-12.6718, -47.4448) construction
  line L5 (-12.6718, -47.4448) -> (-16.194, -45.4113) construction
  line L6 (-16.194, -45.4113) -> (-3.306, -23.0887) construction
  line L7 (-3.306, -23.0887) -> (0.2162, -25.1223) construction
  line L8 (-13.9508, -35.6534) -> (-15.6954, -38.4287) projected
  line L9 (1.25, -57.25) -> (1.25, 1.25) projected
  line L10 (-45.75, 1.25) -> (-45.75, -57.25) projected
  line L11 (-45.75, -57.25) -> (1.25, -57.25) projected
  line L12 (-4.544, -25.3672) -> (-1.0799, -27.3672)
  line L13 (-1.0799, -27.3672) -> (-1.4839, -28.0669)
  line L14 (-1.4839, -28.0669) -> (-3.0232, -27.1781)
  line L15 (-3.0232, -27.1781) -> (-2.2995, -29.4794)
  line L16 (-2.2995, -29.4794) -> (-2.8437, -30.422)
  line L17 (-2.8437, -30.422) -> (-3.4383, -28.3361)
  line L18 (-3.4383, -28.3361) -> (-6.3489, -28.4933)
  line L19 (-6.3489, -28.4933) -> (-5.8261, -27.5877)
  line L20 (-5.8261, -27.5877) -> (-3.6478, -27.5709)
  line L21 (-3.6478, -27.5709) -> (-3.9024, -26.6705)
  line L22 (-3.9024, -26.6705) -> (-4.948, -26.0669)
  line L23 (-4.948, -26.0669) -> (-4.544, -25.3672)
  line L24 (-3.0906, -30.8498) -> (-3.4946, -31.5494)
  line L25 (-3.4946, -31.5494) -> (-5.3718, -30.4656)
  spline S0 degree 2 poles (-5.3718, -30.4656) (-5.8181, -30.208) (-5.9653, -30.1582) knots 0 0 0 1 1 1
  spline S1 degree 2 poles (-5.9653, -30.1582) (-6.2025, -30.0811) (-6.6563, -30.2697) (-6.8255, -30.5627) knots 0 0 0 1 2 2 2
  spline S2 degree 2 poles (-6.8255, -30.5627) (-6.9963, -30.8585) (-6.9287, -31.3023) (-6.6099, -31.5673) (-6.198, -31.8051) knots 0 0 0 1 2 3 3 3
  line L26 (-6.198, -31.8051) -> (-4.2812, -32.9118)
  line L27 (-4.2812, -32.9118) -> (-4.6851, -33.6115)
  line L28 (-4.6851, -33.6115) -> (-6.5043, -32.5612)
  spline S3 degree 2 poles (-6.5043, -32.5612) (-7.1274, -32.2015) (-7.5767, -31.7907) (-7.7552, -31.2828) (-7.6707, -30.6486) (-7.4345, -30.2394) knots 0 0 0 1 2 3 4 4 4
  spline S4 degree 2 poles (-7.4345, -30.2394) (-7.1479, -29.743) (-6.6224, -29.3634) (-6.0858, -29.2754) (-5.8551, -29.3452) knots 0 0 0 1 2 3 3 3
  spline S5 degree 2 poles (-5.8551, -29.3452) (-5.5197, -29.4473) (-4.9388, -29.7827) knots 0 0 0 1 1 1
  line L29 (-4.9388, -29.7827) -> (-3.0906, -30.8498)
  line L30 (-8.5761, -32.3508) -> (-5.112, -34.3508)
  line L31 (-5.112, -34.3508) -> (-5.7598, -35.473)
  spline S6 degree 2 poles (-5.7598, -35.473) (-6.1287, -36.1119) (-6.2928, -36.2742) knots 0 0 0 1 1 1
  spline S7 degree 2 poles (-6.2928, -36.2742) (-6.5416, -36.5283) (-7.2961, -36.6278) (-7.7107, -36.3885) knots 0 0 0 1 2 2 2
  spline S8 degree 2 poles (-7.7107, -36.3885) (-8.0275, -36.2056) (-8.329, -35.7217) (-8.3714, -35.222) (-8.3043, -35.0143) knots 0 0 0 1 2 3 3 3
  spline S9 degree 2 poles (-8.3043, -35.0143) (-8.2112, -34.7371) (-7.9368, -34.2619) knots 0 0 0 1 1 1
  line L32 (-7.9368, -34.2619) -> (-7.6731, -33.8051)
  line L33 (-7.6731, -33.8051) -> (-8.98, -33.0505)
  line L34 (-8.98, -33.0505) -> (-8.5761, -32.3508)
  line L35 (-6.1021, -34.7121) -> (-7.0869, -34.1435)
  line L36 (-7.0869, -34.1435) -> (-7.3079, -34.5263)
  spline S10 degree 2 poles (-7.3079, -34.5263) (-7.5473, -34.9409) (-7.5991, -35.2806) (-7.4582, -35.5732) (-7.3051, -35.6616) knots 0 0 0 1 2 3 3 3
  spline S11 degree 2 poles (-7.3051, -35.6616) (-7.115, -35.7713) (-6.7414, -35.6913) (-6.6106, -35.538) knots 0 0 0 1 2 2 2
  spline S12 degree 2 poles (-6.6106, -35.538) (-6.5152, -35.4276) (-6.2972, -35.0501) knots 0 0 0 1 1 1
  line L37 (-6.2972, -35.0501) -> (-6.1021, -34.7121)
  line L38 (-10.4434, -35.5852) -> (-6.9793, -37.5852)
  line L39 (-6.9793, -37.5852) -> (-7.3711, -38.2638)
  line L40 (-7.3711, -38.2638) -> (-10.5162, -38.3454)
  line L41 (-10.5162, -38.3454) -> (-8.1928, -39.6869)
  line L42 (-8.1928, -39.6869) -> (-8.5662, -40.3338)
  line L43 (-8.5662, -40.3338) -> (-12.0303, -38.3338)
  line L44 (-12.0303, -38.3338) -> (-11.6264, -37.6341)
  line L45 (-11.6264, -37.6341) -> (-8.5436, -37.5446)
  line L46 (-8.5436, -37.5446) -> (-10.8169, -36.2321)
  line L47 (-10.8169, -36.2321) -> (-10.4434, -35.5852)
  line L48 (-12.445, -39.052) -> (-8.9809, -41.052)
  line L49 (-8.9809, -41.052) -> (-9.3848, -41.7516)
  line L50 (-9.3848, -41.7516) -> (-12.8489, -39.7516)
  line L51 (-12.8489, -39.7516) -> (-12.445, -39.052)
  line L52 (-13.2392, -40.4276) -> (-9.7751, -42.4276)
  line L53 (-9.7751, -42.4276) -> (-10.179, -43.1272)
  line L54 (-10.179, -43.1272) -> (-11.7183, -42.2385)
  line L55 (-11.7183, -42.2385) -> (-10.9946, -44.5398)
  line L56 (-10.9946, -44.5398) -> (-11.5388, -45.4824)
  line L57 (-11.5388, -45.4824) -> (-12.1334, -43.3965)
  line L58 (-12.1334, -43.3965) -> (-15.044, -43.5537)
  line L59 (-15.044, -43.5537) -> (-14.5212, -42.6481)
  line L60 (-14.5212, -42.6481) -> (-12.3429, -42.6313)
  line L61 (-12.3429, -42.6313) -> (-12.5976, -41.7309)
  line L62 (-12.5976, -41.7309) -> (-13.6431, -41.1272)
  line L63 (-13.6431, -41.1272) -> (-13.2392, -40.4276)
  line L64 (-29.5367, -45.8895) -> (-29.996, -45.2464)
  spline S13 degree 2 poles (-29.996, -45.2464) (-29.6878, -44.9875) (-29.5837, -44.4239) (-29.7666, -44.1071) knots 0 0 0 1 2 2 2
  spline S14 degree 2 poles (-29.7666, -44.1071) (-29.9617, -43.7691) (-30.4451, -43.5905) (-30.6378, -43.7018) knots 0 0 0 1 2 2 2
  spline S15 degree 2 poles (-30.6378, -43.7018) (-30.7619, -43.7735) (-30.8497, -44.0178) (-30.8094, -44.2339) knots 0 0 0 1 2 2 2
  spline S16 degree 2 poles (-30.8094, -44.2339) (-30.7815, -44.3797) (-30.6367, -44.8805) knots 0 0 0 1 1 1
  spline S17 degree 2 poles (-30.6367, -44.8805) (-30.452, -45.5237) (-30.5242, -45.8681) knots 0 0 0 1 1 1
  spline S18 degree 2 poles (-30.5242, -45.8681) (-30.6249, -46.3523) (-31.0341, -46.5885) knots 0 0 0 1 1 1
  spline S19 degree 2 poles (-31.0341, -46.5885) (-31.3008, -46.7425) (-31.934, -46.7068) (-32.5005, -46.2804) (-32.7307, -45.8818) knots 0 0 0 1 2 3 3 3
  spline S20 degree 2 poles (-32.7307, -45.8818) (-33.1072, -45.2296) (-32.918, -44.2402) (-32.4492, -43.9485) knots 0 0 0 1 2 2 2
  line L65 (-32.4492, -43.9485) -> (-32.0136, -44.6299)
  spline S21 degree 2 poles (-32.0136, -44.6299) (-32.2543, -44.8287) (-32.3186, -45.2601) (-32.1479, -45.5558) knots 0 0 0 1 2 2 2
  spline S22 degree 2 poles (-32.1479, -45.5558) (-31.971, -45.8621) (-31.7478, -45.9621) knots 0 0 0 1 1 1
  spline S23 degree 2 poles (-31.7478, -45.9621) (-31.602, -46.0257) (-31.4673, -45.948) knots 0 0 0 1 1 1
  spline S24 degree 2 poles (-31.4673, -45.948) (-31.3459, -45.8779) (-31.3155, -45.7231) knots 0 0 0 1 1 1
  spline S25 degree 2 poles (-31.3155, -45.7231) (-31.2824, -45.5244) (-31.6321, -44.3638) (-31.658, -43.7275) (-31.3718, -43.1927) (-31.0418, -43.0021) knots 0 0 0 1 2 3 4 4 4
  spline S26 degree 2 poles (-31.0418, -43.0021) (-30.746, -42.8314) (-30.0354, -42.8611) (-29.4328, -43.3194) (-29.1721, -43.7709) knots 0 0 0 1 2 3 3 3
  spline S27 degree 2 poles (-29.1721, -43.7709) (-28.7926, -44.4284) (-28.9928, -45.4839) (-29.5367, -45.8895) knots 0 0 0 1 2 2 2
  line L66 (-33.8357, -43.8337) -> (-34.2396, -43.134)
  line L67 (-34.2396, -43.134) -> (-32.3624, -42.0501)
  spline S28 degree 2 poles (-32.3624, -42.0501) (-31.9162, -41.7925) (-31.7994, -41.6899) knots 0 0 0 1 1 1
  spline S29 degree 2 poles (-31.7994, -41.6899) (-31.6141, -41.523) (-31.5504, -41.0357) (-31.7197, -40.7426) knots 0 0 0 1 2 2 2
  spline S30 degree 2 poles (-31.7197, -40.7426) (-31.8904, -40.4469) (-32.3086, -40.2835) (-32.6975, -40.427) (-33.1094, -40.6649) knots 0 0 0 1 2 3 3 3
  line L68 (-33.1094, -40.6649) -> (-35.0262, -41.7716)
  line L69 (-35.0262, -41.7716) -> (-35.4302, -41.0719)
  line L70 (-35.4302, -41.0719) -> (-33.611, -40.0216)
  spline S31 degree 2 poles (-33.611, -40.0216) (-32.9879, -39.6618) (-32.4075, -39.4781) (-31.8784, -39.5775) (-31.3714, -39.9677) (-31.1351, -40.377) knots 0 0 0 1 2 3 4 4 4
  spline S32 degree 2 poles (-31.1351, -40.377) (-30.8486, -40.8734) (-30.7825, -41.5182) (-30.9746, -42.0269) (-31.1505, -42.1918) knots 0 0 0 1 2 3 3 3
  spline S33 degree 2 poles (-31.1505, -42.1918) (-31.4066, -42.4312) (-31.9875, -42.7666) knots 0 0 0 1 1 1
  line L71 (-31.9875, -42.7666) -> (-33.8357, -43.8337)
  line L72 (-32.3929, -38.3326) -> (-35.857, -40.3326)
  line L73 (-35.857, -40.3326) -> (-36.5049, -39.2104)
  spline S34 degree 2 poles (-36.5049, -39.2104) (-36.8738, -38.5715) (-36.9323, -38.3483) knots 0 0 0 1 1 1
  spline S35 degree 2 poles (-36.9323, -38.3483) (-37.0279, -38.0057) (-36.7369, -37.3025) (-36.3223, -37.0632) knots 0 0 0 1 2 2 2
  spline S36 degree 2 poles (-36.3223, -37.0632) (-36.0055, -36.8803) (-35.4357, -36.8611) (-34.9817, -37.0743) (-34.8354, -37.2362) knots 0 0 0 1 2 3 3 3
  spline S37 degree 2 poles (-34.8354, -37.2362) (-34.642, -37.4554) (-34.3676, -37.9307) knots 0 0 0 1 1 1
  line L74 (-34.3676, -37.9307) -> (-34.1038, -38.3875)
  line L75 (-34.1038, -38.3875) -> (-32.7969, -37.6329)
  line L76 (-32.7969, -37.6329) -> (-32.3929, -38.3326)
  line L77 (-35.6748, -39.2945) -> (-34.69, -38.7259)
  line L78 (-34.69, -38.7259) -> (-34.911, -38.343)
  spline S38 degree 2 poles (-34.911, -38.343) (-35.1504, -37.9285) (-35.4187, -37.7138) (-35.7425, -37.6895) (-35.8956, -37.7779) knots 0 0 0 1 2 3 3 3
  spline S39 degree 2 poles (-35.8956, -37.7779) (-36.0857, -37.8877) (-36.2032, -38.2512) (-36.1358, -38.4411) knots 0 0 0 1 2 2 2
  spline S40 degree 2 poles (-36.1358, -38.4411) (-36.0879, -38.579) (-35.87, -38.9565) knots 0 0 0 1 1 1
  line L79 (-35.87, -38.9565) -> (-35.6748, -39.2945)
  line L80 (-34.2572, -35.1035) -> (-37.7213, -37.1035)
  line L81 (-37.7213, -37.1035) -> (-38.3692, -35.9813)
  spline S41 degree 2 poles (-38.3692, -35.9813) (-38.7381, -35.3424) (-38.7966, -35.1191) knots 0 0 0 1 1 1
  spline S42 degree 2 poles (-38.7966, -35.1191) (-38.8923, -34.7766) (-38.6012, -34.0734) (-38.1867, -33.8341) knots 0 0 0 1 2 2 2
  spline S43 degree 2 poles (-38.1867, -33.8341) (-37.8698, -33.6512) (-37.3, -33.632) (-36.8461, -33.8451) (-36.6997, -34.0071) knots 0 0 0 1 2 3 3 3
  spline S44 degree 2 poles (-36.6997, -34.0071) (-36.5063, -34.2263) (-36.2319, -34.7016) knots 0 0 0 1 1 1
  line L82 (-36.2319, -34.7016) -> (-35.9682, -35.1584)
  line L83 (-35.9682, -35.1584) -> (-34.6612, -34.4038)
  line L84 (-34.6612, -34.4038) -> (-34.2572, -35.1035)
  line L85 (-37.5392, -36.0654) -> (-36.5543, -35.4968)
  line L86 (-36.5543, -35.4968) -> (-36.7754, -35.1139)
  spline S45 degree 2 poles (-36.7754, -35.1139) (-37.0147, -34.6994) (-37.283, -34.4847) (-37.6068, -34.4604) (-37.76, -34.5488) knots 0 0 0 1 2 3 3 3
  spline S46 degree 2 poles (-37.76, -34.5488) (-37.9501, -34.6586) (-38.0676, -35.0221) (-38.0002, -35.212) knots 0 0 0 1 2 2 2
  spline S47 degree 2 poles (-38.0002, -35.212) (-37.9523, -35.3498) (-37.7343, -35.7274) knots 0 0 0 1 1 1
  line L87 (-37.7343, -35.7274) -> (-37.5392, -36.0654)
  line L88 (-36.1216, -31.8744) -> (-39.5857, -33.8744)
  line L89 (-39.5857, -33.8744) -> (-41.0689, -31.3053)
  line L90 (-41.0689, -31.3053) -> (-40.4828, -30.9669)
  line L91 (-40.4828, -30.9669) -> (-39.4035, -32.8363)
  line L92 (-39.4035, -32.8363) -> (-38.6352, -32.3927)
  line L93 (-38.6352, -32.3927) -> (-39.6397, -30.6527)
  line L94 (-39.6397, -30.6527) -> (-39.0536, -30.3143)
  line L95 (-39.0536, -30.3143) -> (-38.049, -32.0542)
  line L96 (-38.049, -32.0542) -> (-37.1117, -31.5131)
  line L97 (-37.1117, -31.5131) -> (-38.2291, -29.5777)
  line L98 (-38.2291, -29.5777) -> (-37.6429, -29.2393)
  line L99 (-37.6429, -29.2393) -> (-36.1216, -31.8744)
  line L100 (-37.9966, -28.6268) -> (-41.4316, -30.61)
  line L101 (-41.4316, -30.61) -> (-41.8356, -29.9103)
  line L102 (-41.8356, -29.9103) -> (-38.9867, -28.2655)
  line L103 (-38.9867, -28.2655) -> (-39.9913, -26.5255)
  line L104 (-39.9913, -26.5255) -> (-39.4051, -26.1871)
  line L105 (-39.4051, -26.1871) -> (-37.9966, -28.6268)
  line L106 (-40.1429, -24.9092) -> (-43.0209, -26.5708)
  line L107 (-43.0209, -26.5708) -> (-42.4279, -27.5979)
  line L108 (-42.4279, -27.5979) -> (-43.014, -27.9363)
  line L109 (-43.014, -27.9363) -> (-44.6024, -25.1851)
  line L110 (-44.6024, -25.1851) -> (-44.0163, -24.8466)
  line L111 (-44.0163, -24.8466) -> (-43.4248, -25.8711)
  line L112 (-43.4248, -25.8711) -> (-40.5469, -24.2095)
  line L113 (-40.5469, -24.2095) -> (-40.1429, -24.9092)
  point P0 (0, 0)
  point P1 (-34.75, -34.25)
  point P2 (-9.75, -34.25)
  dimension "d21" = 25.7759
  dimension "d22" = 25.7759
  dimension "d23" = 4.0671
  dimension "d24" = 4.0671
  dimension "d25" = 30
  dimension "d26" = 30
  dimension "d27" = 23
  dimension "d28" = 11
  dimension "d29" = 11
  constraints: 2 midpoint, 1 horizontal alignment, 4 other
  measures "d21" distance of L1.end L2.end
  measures "d22" distance of L4.start L4.end
  measures "d23" distance of L4.end L5.end
  measures "d24" distance of L0.end L1.end
  measures "d25" angle of L6 L9
  measures "d26" angle of L10 L2
  measures "d27" distance from line of L11 point (-9.75, -34.25)
  measures "d28" distance from line of L9 point (-9.75, -34.25)
  measures "d29" distance from line of point (-34.75, -34.25) L10
extrude "Extrusion7" cut sketch "Skizze9" against normal blind 0.4
equation "\"d4\" = d3"
equation "\"d6\" = d5"
equation "\"d22\" = d21"
equation "\"d24\" = d23"
equation "\"d26\" = d25"
equation "\"d29\" = d28"
body "Solid1"
